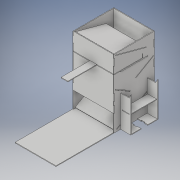
# Autodesk Inventor part: Full Tower
Saved by Autodesk Inventor 2017 (Build 210142000, 142)
## iProperties
Created: 2017-03-26
Part Number: Full Tower
Material: Generic
Document SubType Name: Modeling
Designer: Bearbiever
Density: 1 g/cm^3
Appearance: Default
Author: Bearbiever
Autodesk Inventor part; units mm, degrees
ref_plane "YZ Plane" through (0, 0, 0) normal (1, 0, 0) x (0, 1, 0)
ref_plane "XZ Plane" through (0, 0, 0) normal (0, 1, 0) x (-1, 0, 0)
ref_plane "XY Plane" through (0, 0, 0) normal (0, 0, 1) x (1, 0, 0)
sketch "Sketch15" plane through (0, 0, 0) normal (1, 0, 0) x (0, 1, 0)
  line L0 (254, 0) -> (254, 152.4)
  line L1 (190.4803, 152.4) -> (190.4803, 46.99)
  line L2 (195.0007, 142.6426) -> (201.7101, 142.6426) construction
  line L3 (201.7101, 142.6426) -> (201.7101, 48.7112) construction
  line L4 (201.7101, 48.7112) -> (195.0007, 48.7112) construction
  line L5 (195.0007, 48.7112) -> (195.0007, 142.6426) construction
  line L6 (190.4803, 152.4) -> (190.4803, 273.05)
  line L7 (6.35, 141.4015) -> (75.2882, 21.997)
  line L8 (136.614, 147.0706) -> (104.864, 92.078)
  line L9 (247.1811, 145.8462) -> (216.6784, 32.0086)
  line L10 (175.7069, 3.6254) -> (137.6069, 69.6166)
  line L11 (190.4803, 44.45) -> (203.1803, 44.45)
  line L12 (137.6069, 69.6166) -> (139.8066, 70.8866)
  line L13 (139.8066, 70.8866) -> (177.9066, 4.8954)
  line L14 (104.864, 92.078) -> (107.3637, 90.6348)
  line L15 (0, 152.4) -> (0.1917, 152.5107)
  line L16 (190.4803, 44.45) -> (187.9403, 44.45)
  line L17 (187.9403, 127) -> (187.9403, 273.05)
  line L18 (187.9403, 273.05) -> (190.4803, 273.05)
  line L19 (203.1803, 44.45) -> (203.1803, 46.99)
  line L20 (203.1803, 46.99) -> (190.4803, 46.99)
  line L21 (216.6784, 32.0086) -> (219.1318, 31.3512)
  line L22 (219.1318, 31.3512) -> (249.6345, 145.1888)
  line L23 (187.9403, 127) -> (185.4003, 127)
  line L24 (185.4003, 127) -> (185.4003, 25.4)
  line L25 (185.4003, 25.4) -> (187.9403, 25.4)
  line L26 (187.9403, 25.4) -> (187.9403, 44.45)
  line L27 (254, 0) -> (228.6, 0)
  line L28 (228.6, 0) -> (228.6, 2.54)
  line L29 (228.6, 2.54) -> (203.2, 2.54)
  line L30 (203.2, 2.54) -> (203.2, 0)
  line L31 (165.1, 0) -> (165.1, 2.54)
  line L32 (165.1, 2.54) -> (139.7, 2.54)
  line L33 (139.7, 2.54) -> (139.7, 0)
  line L34 (139.7, 0) -> (76.2, 0)
  line L35 (76.2, 0) -> (76.2, 2.54)
  line L36 (76.2, 2.54) -> (50.8, 2.54)
  line L37 (50.8, 2.54) -> (50.8, 0)
  line L38 (228.6, 0) -> (254, 0)
  line L39 (76.2, 0) -> (139.7, 0)
  line L40 (254, 152.4) -> (241.3, 152.4)
  line L41 (241.3, 152.4) -> (241.3, 149.86)
  line L42 (241.3, 149.86) -> (215.9, 149.86)
  line L43 (215.9, 149.86) -> (215.9, 152.4)
  line L44 (254, 152.4) -> (241.3, 152.4)
  line L45 (127, 152.4) -> (127, 149.86)
  line L46 (127, 149.86) -> (101.6, 149.86)
  line L47 (101.6, 149.86) -> (101.6, 152.4)
  line L48 (101.6, 152.4) -> (88.9, 152.4)
  line L49 (88.9, 152.4) -> (88.9, 149.86)
  line L50 (88.9, 149.86) -> (63.5, 149.86)
  line L51 (63.5, 149.86) -> (63.5, 152.4)
  line L52 (63.5, 152.4) -> (38.1, 152.4)
  line L53 (63.5, 152.4) -> (0, 152.4)
  line L54 (101.6, 152.4) -> (88.9, 152.4)
  line L55 (0, 152.4) -> (0, 127)
  line L56 (0, 127) -> (2.54, 127)
  line L57 (2.54, 127) -> (2.54, 88.9)
  line L58 (2.54, 88.9) -> (0, 88.9)
  line L59 (0, 88.9) -> (0, 63.5)
  line L60 (0, 63.5) -> (2.54, 63.5)
  line L61 (2.54, 63.5) -> (2.54, 25.4)
  line L62 (2.54, 25.4) -> (0, 25.4)
  line L63 (0, 152.4) -> (0, 127)
  line L64 (0, 88.9) -> (0, 63.5)
  line L65 (75.2882, 21.997) -> (77.4879, 23.267)
  line L66 (8.5497, 142.6715) -> (6.35, 141.4015)
  line L67 (8.5497, 142.6715) -> (77.4879, 23.267)
  line L68 (139.1137, 145.6275) -> (107.3637, 90.6348)
  line L69 (177.9066, 4.8954) -> (175.7069, 3.6254)
  line L70 (247.1811, 145.8462) -> (249.6345, 145.1888)
  line L71 (136.614, 147.0706) -> (139.1137, 145.6275)
  line L72 (127, 152.4) -> (187.9403, 152.4)
  line L73 (0, 25.4) -> (0, 0)
  line L74 (0, 0) -> (50.8, 0)
  line L75 (215.9, 152.4) -> (190.4803, 152.4)
  line L76 (203.2, 0) -> (165.1, 0)
  dimension "d39" = 254
  dimension "d40" = 152.4
  dimension "d42" = 120.65
  dimension "d49" = 12.7
  dimension "d53" = 2.54
  dimension "d56" = 2.54
  dimension "d57" = 2.54
  dimension "d58" = 2.54
  dimension "d59" = 2.54
  dimension "d60" = 101.6
  dimension "d62" = 25.4
  dimension "d65" = 2.54
  dimension "d66" = 25.4
  dimension "d67" = 38.1
  dimension "d68" = 2.54
  dimension "d69" = 25.4
  dimension "d70" = 63.5
  dimension "d71" = 2.54
  dimension "d72" = 25.4
  dimension "d73" = 12.7
  dimension "d74" = 2.54
  dimension "d75" = 25.4
  dimension "d80" = 2.54
  dimension "d81" = 25.4
  dimension "d82" = 12.7
  dimension "d83" = 2.54
  dimension "d84" = 25.4
  dimension "d85" = 25.4
  dimension "d86" = 25.4
  dimension "d87" = 2.54
  dimension "d88" = 38.1
  dimension "d89" = 25.4
  dimension "d90" = 2.54
  dimension "d91" = 38.1
  dimension "d94" = 6.35
  dimension "d95" = 30
  dimension "d96" = 76.2
  dimension "d98" = 63.5
  dimension "d99" = 25.4
  dimension "d100" = 50.8
  dimension "d101" = 2.54
  dimension "d102" = 2.54
  dimension "d103" = 2.54
  constraints: 154 end point, 47 perpendicular, 14 parallel, 9 horizontal, 7 point on line, 5 vertical
  measures "d39" distance of L15.start L0.end
  measures "d40" distance of L0.end L0.start
  measures "d42" distance of L1.start L6.end
  measures "d49" distance of L11.start L11.end
  measures "d53" distance of L10.end L12.end
  measures "d56" distance of L16.end L11.start
  measures "d57" distance of L11.end L19.end
  measures "d58" distance of L9.end L21.end
  measures "d59" distance of L25.end L24.end
  measures "d60" distance of L24.end L23.end
  measures "d62" distance of L0.start L27.end
  measures "d65" distance of L27.end L28.end
  measures "d66" distance of L28.end L29.end
  measures "d67" distance of L30.end L31.start
  measures "d68" distance of L31.start L31.end
  measures "d69" distance of L31.end L32.end
  measures "d70" distance of L33.end L34.end
  measures "d71" distance of L34.end L35.end
  measures "d72" distance of L35.end L36.end
  measures "d73" distance of L0.end L40.end
  measures "d74" distance of L40.end L41.end
  measures "d75" distance of L41.end L42.end
  measures "d80" distance of L45.start L45.end
  measures "d81" distance of L45.end L46.end
  measures "d82" distance of L47.end L48.end
  measures "d83" distance of L48.end L49.end
  measures "d84" distance of L49.end L50.end
  measures "d85" distance of L51.end L52.end
  measures "d86" distance of L15.start L55.end
  measures "d87" distance of L55.end L56.end
  measures "d88" distance of L56.end L57.end
  measures "d89" distance of L58.end L59.end
  measures "d90" distance of L59.end L60.end
  measures "d91" distance of L60.end L61.end
  measures "d94" distance from line of L55 L7.start
  measures "d95" angle of L55 L7
  measures "d96" distance between parallel lines of L69 L12
  measures "d98" distance between parallel lines of L14 L71
  measures "d99" distance of L73.end L62.end
  measures "d100" distance of L73.end L37.end
  measures "d101" distance of L61.end L62.end
  measures "d102" distance of L36.end L37.end
  measures "d103" distance of L32.end L33.end
extrude "Extrusion10" add sketch "Sketch15" along normal blind 2.54 contours L27 L28 L29 L30 L76 L31 L32 L33 L34 L35 L36 L37 L74 L73 L62 L61 L60 L59 L58 L57 L56 L55 L53 L52 L51 L50 L49 L48 L47 L46 L45 L72 L17 L23 L24 L25 L26 L16 L11 L19 L20 L1 L75 L43 L42 L41 L40 L0
sketch "Sketch16" plane through (0, 0, 0) normal (0, 0, -1) x (-1, 0, 0)
  line L0 (0, 0) -> (147.32, 0)
  line L1 (0, 0) -> (0, 50.8)
  line L2 (0, 50.8) -> (-2.54, 50.8)
  line L3 (-2.54, 50.8) -> (-2.54, 76.2)
  line L4 (-2.54, 76.2) -> (0, 76.2)
  line L5 (0, 139.7) -> (-2.54, 139.7) projected
  line L6 (0, 76.2) -> (0, 139.7)
  line L7 (0, 139.7) -> (-2.54, 139.7)
  line L8 (0, 165.1) -> (-2.54, 165.1) projected
  line L9 (-2.54, 139.7) -> (-2.54, 165.1)
  line L10 (-2.54, 165.1) -> (0, 165.1)
  line L11 (0, 165.1) -> (0, 203.2) projected
  line L12 (0, 165.1) -> (0, 203.2)
  line L13 (0, 203.2) -> (-2.54, 203.2)
  line L14 (-2.54, 203.2) -> (-2.54, 228.6) projected
  line L15 (-2.54, 203.2) -> (-2.54, 228.6)
  line L16 (-2.54, 228.6) -> (0, 228.6)
  line L17 (0, 254) -> (-2.54, 254) projected
  line L18 (0, 228.6) -> (0, 254)
  line L19 (0, 254) -> (147.32, 254)
  line L20 (147.32, 0) -> (147.32, 50.8)
  line L21 (147.32, 50.8) -> (149.86, 50.8)
  line L22 (149.86, 50.8) -> (149.86, 76.2)
  line L23 (149.86, 76.2) -> (147.32, 76.2)
  line L24 (147.32, 76.2) -> (147.32, 139.7)
  line L25 (147.32, 139.7) -> (149.86, 139.7)
  line L26 (149.86, 139.7) -> (149.86, 165.1)
  line L27 (149.86, 165.1) -> (147.32, 165.1)
  line L28 (147.32, 165.1) -> (147.32, 203.2)
  line L29 (147.32, 203.2) -> (149.86, 203.2)
  line L30 (149.86, 203.2) -> (149.86, 228.6)
  line L31 (149.86, 228.6) -> (147.32, 228.6)
  line L32 (147.32, 228.6) -> (147.32, 254)
  dimension "d106" = 147.32
  dimension "d107" = 147.32
  dimension "d108" = 50.8
  dimension "d109" = 2.54
  dimension "d110" = 25.4
  dimension "d111" = 2.54
  constraints: 56 end point, 18 perpendicular, 12 point on line, 2 vertical, 1 horizontal
  measures "d106" distance of L0.start L0.end
  measures "d107" distance of L17.start L19.end
  measures "d108" distance of L0.end L20.end
  measures "d109" distance of L20.end L21.end
  measures "d110" distance of L21.end L22.end
  measures "d111" distance of L24.end L25.end
extrude "Extrusion11" add sketch "Sketch16" against normal blind 2.54 separate body
sketch "Sketch19" plane through (-149.86, 203.2, 0) normal (-1, 0, 0) x (0, 0, 1)
  line L0 (0, 50.8) -> (152.4, 50.8) projected
  line L1 (152.4, 50.8) -> (0, 50.8)
  line L2 (0, 0) -> (0, 25.4) projected
  line L3 (0, 50.8) -> (0, 25.4)
  line L4 (2.54, 50.8) -> (2.54, 25.4) projected
  line L5 (0, 25.4) -> (2.54, 25.4)
  line L6 (2.54, 25.4) -> (2.54, 0)
  line L7 (2.54, 0) -> (0, 0)
  line L8 (0, -38.1) -> (0, -63.5) projected
  line L9 (0, 0) -> (0, -38.1)
  line L10 (0, -38.1) -> (2.54, -38.1)
  line L11 (2.54, -127) -> (2.54, -63.5) projected
  line L12 (2.54, -38.1) -> (2.54, -63.5)
  line L13 (2.54, -63.5) -> (0, -63.5)
  line L14 (0, -127) -> (0, -152.4) projected
  line L15 (0, -63.5) -> (0, -127)
  line L16 (2.54, -152.4) -> (2.54, -127) projected
  line L17 (2.54, -127) -> (2.54, -152.4)
  line L18 (2.54, -152.4) -> (0, -152.4)
  line L19 (0, -203.2) -> (25.4, -203.2)
  line L20 (63.5, -200.66) -> (25.4, -200.66) projected
  line L21 (25.4, -203.2) -> (25.4, -200.66)
  line L22 (25.4, -200.66) -> (63.5, -200.66)
  line L23 (63.5, -200.66) -> (63.5, -203.2)
  line L24 (63.5, -203.2) -> (88.9, -203.2)
  line L25 (88.9, -203.2) -> (88.9, -200.66)
  line L26 (127, -203.2) -> (127, -200.66) projected
  line L27 (88.9, -200.66) -> (127, -200.66)
  line L28 (127, -200.66) -> (127, -203.2)
  line L29 (127, -203.2) -> (152.4, -203.2)
  line L30 (152.4, -203.2) -> (152.4, -139.7)
  line L31 (149.86, -139.7) -> (152.4, -139.7) projected
  line L32 (152.4, -139.7) -> (149.86, -139.7)
  line L33 (149.86, -139.7) -> (149.86, -114.3)
  line L34 (152.4, -101.6) -> (152.4, -114.3) projected
  line L35 (149.86, -114.3) -> (152.4, -114.3)
  line L36 (152.4, -114.3) -> (152.4, -101.6)
  line L37 (152.4, -101.6) -> (149.86, -101.6)
  line L38 (152.4, -76.2) -> (149.86, -76.2) projected
  line L39 (149.86, -101.6) -> (149.86, -76.2)
  line L40 (149.86, -76.2) -> (152.4, -76.2)
  line L41 (127, -15.2597) -> (152.4, -15.2597) projected
  line L42 (152.4, -76.2) -> (152.4, -15.2597)
  line L43 (152.4, -15.2597) -> (127, -15.2597)
  line L44 (25.4, -17.7997) -> (127, -17.7997) projected
  line L45 (127, -15.2597) -> (127, -17.7997)
  line L46 (127, -17.7997) -> (25.4, -17.7997)
  line L47 (25.4, -17.7997) -> (25.4, -15.2597)
  line L48 (25.4, -15.2597) -> (44.45, -15.2597)
  line L49 (44.45, -0.0197) -> (44.45, -15.2597) projected
  line L50 (44.45, -15.2597) -> (44.45, -0.0197)
  line L51 (44.45, -0.0197) -> (46.99, -0.0197)
  line L52 (46.99, -12.7197) -> (46.99, -0.0197) projected
  line L53 (46.99, -0.0197) -> (46.99, -12.7197)
  line L54 (152.4, 12.7) -> (152.4, -12.7197) projected
  line L55 (46.99, -12.7197) -> (152.4, -12.7197)
  line L56 (152.4, -12.7197) -> (152.4, 12.7)
  line L57 (149.86, 12.7) -> (152.4, 12.7) projected
  line L58 (152.4, 12.7) -> (149.86, 12.7)
  line L59 (149.86, 12.7) -> (149.86, 38.1)
  line L60 (149.86, 38.1) -> (152.4, 38.1)
  line L61 (152.4, 38.1) -> (152.4, 50.8)
  line L62 (31.3512, 15.9318) -> (145.1888, 46.4345)
  line L63 (145.1888, 46.4345) -> (145.8462, 43.9811)
  line L64 (31.3512, 15.9318) -> (32.0086, 13.4784) projected
  line L65 (145.8462, 43.9811) -> (32.0086, 13.4784)
  line L66 (32.0086, 13.4784) -> (31.3512, 15.9318)
  line L67 (4.8954, -25.2934) -> (70.8866, -63.3934) projected
  line L68 (4.8954, -25.2934) -> (70.8866, -63.3934)
  line L69 (70.8866, -63.3934) -> (69.6166, -65.5931) projected
  line L70 (70.8866, -63.3934) -> (69.6166, -65.5931)
  line L71 (69.6166, -65.5931) -> (3.6254, -27.4931) projected
  line L72 (69.6166, -65.5931) -> (3.6254, -27.4931)
  line L73 (3.6254, -27.4931) -> (4.8954, -25.2934) projected
  line L74 (3.6254, -27.4931) -> (4.8954, -25.2934)
  line L75 (147.0706, -66.586) -> (145.6275, -64.0863) projected
  line L76 (145.6275, -64.0863) -> (147.0706, -66.586)
  line L77 (147.0706, -66.586) -> (92.078, -98.336)
  line L78 (92.078, -98.336) -> (90.6348, -95.8363)
  line L79 (90.6348, -95.8363) -> (145.6275, -64.0863)
  line L80 (23.267, -125.7121) -> (142.6715, -194.6503) projected
  line L81 (23.267, -125.7121) -> (21.997, -127.9118)
  line L82 (141.4015, -196.85) -> (21.997, -127.9118) projected
  line L83 (21.997, -127.9118) -> (141.4015, -196.85)
  line L84 (141.4015, -196.85) -> (142.6715, -194.6503)
  line L85 (142.6715, -194.6503) -> (23.267, -125.7121)
  line L86 (0, -152.4) -> (0, -203.2)
  dimension "d157" = 25.4
  dimension "d158" = 2.54
  dimension "d159" = 2.54
  constraints: 122 end point, 41 perpendicular, 12 collinear, 11 point on line, 2 horizontal, 2 vertical
  measures "d157" distance of L31.start L33.end
  measures "d158" distance of L62.end L63.end
  measures "d159" distance of L67.end L69.end
extrude "Extrusion12" add sketch "Sketch19" against normal blind 2.54 separate body contours L0 L4 L5 L3 | L0 L61 L60 L59 L57 L54 L55 L52 L51 L49 L48 L47 L44 L45 L41 L42 L38 L39 L37 L34 L35 L33 L31 L30 L29 L26 L27 L25 L24 L23 L20 L21 L19 L86 L18 L16 L11 L12 L10 L9 L7 L6 L4
sketch "Sketch20" plane through (-149.86, 187.9403, 152.4) normal (0, 1, 0) x (1, 0, 0)
  line L0 (152.4, 127) -> (152.4, 25.4) projected
  line L1 (0, 0) -> (0, 107.95)
  line L2 (0, 107.95) -> (152.4, 107.95)
  line L3 (152.4, 107.95) -> (152.4, 0)
  line L4 (88.9, 0) -> (88.9, -107.95)
  line L5 (88.9, -107.95) -> (63.5, -107.95)
  line L6 (63.5, -107.95) -> (63.5, 0)
  line L7 (152.4, 0) -> (88.9, 0)
  line L8 (63.5, 0) -> (0, 0)
  point P0 (149.86, 152.4)
  dimension "d163" = 107.95
  dimension "d164" = 152.4
  dimension "d165" = 107.95
  dimension "d166" = 25.4
  dimension "d167" = 63.5
  constraints: 16 end point, 8 perpendicular, 1 point on line, 1 vertical
  measures "d163" distance of L1.start L1.end
  measures "d164" distance of L1.end L2.end
  measures "d165" distance of L4.start L4.end
  measures "d166" distance of L4.end L5.end
  measures "d167" distance of L1.start L6.end
extrude "Extrusion13" add sketch "Sketch20" along normal blind 2.54 separate body
sketch "Sketch21" plane through (0, 187.9403, 44.45) normal (0, 0, 1) x (1, 0, 0)
  line L0 (2.54, 15.24) -> (2.54, 0) projected
  line L1 (2.54, 2.5499) -> (-149.86, 2.5499)
  line L2 (-149.86, 2.5499) -> (-149.86, 15.2499)
  line L3 (-149.86, 15.2499) -> (2.54, 15.2499)
  line L4 (2.54, 15.2499) -> (2.54, 2.5499)
  point P0 (0, -187.9403)
  dimension "d170" = 152.4
  dimension "d171" = 12.7
  constraints: 8 end point, 2 parallel, 1 horizontal, 1 perpendicular, 1 point on line
  measures "d170" distance of L2.end L3.end
  measures "d171" distance of L1.end L2.end
extrude "Extrusion14" add sketch "Sketch21" along normal blind 2.54 separate body
sketch "Sketch23" plane through (-149.86, 241.3, 152.4) normal (0, 0, 1) x (1, 0, 0)
  line L0 (149.86, 12.7) -> (149.86, 0) projected
  line L1 (2.54, 12.7) -> (149.86, 12.7)
  line L2 (149.86, 12.7) -> (149.86, 0)
  line L3 (149.86, 0) -> (152.4, 0)
  line L4 (152.4, 0) -> (152.4, -25.4)
  line L5 (152.4, -25.4) -> (149.86, -25.4)
  line L6 (149.86, -114.3) -> (152.4, -114.3) projected
  line L7 (149.86, -25.4) -> (149.86, -114.3)
  line L8 (149.86, -114.3) -> (152.4, -114.3)
  line L9 (152.4, -114.3) -> (152.4, -139.7)
  line L10 (149.86, -139.7) -> (149.86, -152.4) projected
  line L11 (152.4, -139.7) -> (149.86, -139.7)
  line L12 (149.86, -139.7) -> (149.86, -152.4)
  line L13 (149.86, -152.4) -> (152.4, -152.4) projected
  line L14 (149.86, -152.4) -> (152.4, -152.4)
  line L15 (152.4, -177.8) -> (152.4, -241.3) projected
  line L16 (152.4, -152.4) -> (152.4, -177.8)
  line L17 (149.86, -177.8) -> (149.86, -241.3) projected
  line L18 (152.4, -177.8) -> (149.86, -177.8)
  line L19 (2.54, -177.8) -> (0, -177.8)
  line L20 (0, -177.8) -> (0, -152.4)
  line L21 (0, -152.4) -> (2.54, -152.4)
  line L22 (2.54, -152.4) -> (2.54, -139.7)
  line L23 (2.54, -139.7) -> (0, -139.7)
  line L24 (0, -114.3) -> (0, -53.3597) projected
  line L25 (0, -139.7) -> (0, -114.3)
  line L26 (0, -114.3) -> (2.54, -114.3)
  line L27 (2.54, -25.4) -> (2.54, -50.8197) projected
  line L28 (2.54, -114.3) -> (2.54, -25.4)
  line L29 (2.54, -25.4) -> (0, -25.4)
  line L30 (0, 0) -> (0, 12.7) projected
  line L31 (0, -25.4) -> (0, 0)
  line L32 (0, 0) -> (2.54, 0)
  line L33 (2.54, 0) -> (2.54, 12.7)
  line L34 (63.5, -53.3597) -> (63.5, -50.8197) projected
  line L35 (88.9, -50.8197) -> (152.4, -50.8197) projected
  line L36 (63.5, -53.3597) -> (88.9, -53.3597)
  line L37 (88.9, -53.3597) -> (88.9, -50.8197)
  line L38 (88.9, -50.8197) -> (63.5, -50.8197)
  line L39 (63.5, -50.8197) -> (63.5, -53.3597)
  line L40 (2.54, -177.8) -> (149.86, -177.8)
  point P0 (149.86, -196.85)
  dimension "d175" = 2.54
  dimension "d176" = 19.05
  constraints: 60 end point, 18 perpendicular, 4 point on line, 2 collinear, 2 horizontal, 2 parallel
  measures "d175" distance of L0.end L3.end
  measures "d176" distance of L17.start point (149.86, -196.85)
sketch "Sketch22" plane through (0, 247.1811, 145.8462) normal (0, 0.9659258, -0.258819) x (1, 0, 0)
  line L0 (0, 117.8533) -> (2.54, 117.8533) projected
  line L1 (0, 0) -> (2.54, 0) projected
  line L2 (2.54, 0) -> (-149.86, 0)
  line L3 (-149.86, 0) -> (-149.86, 117.8533)
  line L4 (-149.86, 117.8533) -> (2.54, 117.8533)
  line L5 (2.54, 117.8533) -> (2.54, 0)
  point P0 (0, 204.8517)
  dimension "d174" = 152.4
  constraints: 8 end point, 2 parallel, 1 horizontal, 1 perpendicular
  measures "d174" distance of L3.end L4.end
extrude "Extrusion15" add sketch "Sketch22" along normal blind 2.54 separate body
extrude "Extrusion16" add sketch "Sketch23" against normal blind 2.54 separate body
sketch "Sketch24" plane through (-149.86, 177.9066, 4.8954) normal (0, -0.8660254, -0.5) x (1, 0, 0)
  line L0 (0, 0) -> (2.54, 0) projected
  line L1 (0, 76.2) -> (2.54, 76.2) projected
  line L2 (0, 0) -> (0, 76.2)
  line L3 (152.4, 76.2) -> (152.4, 0) projected
  line L4 (0, 76.2) -> (152.4, 76.2)
  line L5 (0, 30.1632) -> (152.4, 30.1632) projected
  line L6 (152.4, 76.2) -> (152.4, 0)
  line L7 (2.54, 0) -> (2.54, -2.1623)
  line L8 (2.54, -2.1623) -> (149.86, -2.1623)
  line L9 (149.86, -2.1623) -> (149.86, 0)
  line L10 (0, 0) -> (2.54, 0)
  line L11 (149.86, 0) -> (152.4, 0)
  point P0 (149.86, 84.7137)
  dimension "d182" = 152.4
  dimension "d183" = 152.4
  dimension "d184" = 147.32
  constraints: 16 end point, 5 perpendicular, 3 vertical, 1 parallel
  measures "d182" distance of L0.start L3.end
  measures "d183" distance of L1.start L3.start
  measures "d184" distance of L7.end L8.end
extrude "Extrusion17" add sketch "Sketch24" along normal blind 2.54 separate body
sketch "Sketch25" plane through (-149.86, 107.3637, 90.6348) normal (0, -0.8660254, 0.5) x (1, 0, 0)
  line L0 (152.4, 63.5) -> (152.4, 0) projected
  line L1 (152.4, 0) -> (152.4, 63.5)
  line L2 (152.4, 0) -> (0, 0)
  line L3 (0, 63.5) -> (2.54, 63.5) projected
  line L4 (0, 0) -> (0, 63.5)
  line L5 (149.86, 63.5) -> (149.86, 66.04)
  line L6 (149.86, 66.04) -> (2.54, 66.04)
  line L7 (2.54, 66.04) -> (2.54, 63.5)
  line L8 (0, 63.5) -> (2.54, 63.5)
  line L9 (149.86, 63.5) -> (152.4, 63.5)
  point P0 (149.86, -132.1739)
  dimension "d187" = 152.4
  dimension "d188" = 152.4
  dimension "d189" = 2.54
  dimension "d190" = 147.32
  constraints: 16 end point, 2 perpendicular, 1 collinear, 1 horizontal, 1 vertical
  measures "d187" distance of L0.end L2.end
  measures "d188" distance of L3.start L0.start
  measures "d189" distance of L5.start L5.end
  measures "d190" distance of L5.end L6.end
extrude "Extrusion18" add sketch "Sketch25" along normal blind 2.54 separate body
sketch "Sketch26" plane through (0, 6.35, 141.4015) normal (0, 0.8660254, 0.5) x (1, 0, 0)
  line L0 (2.54, 137.8764) -> (2.54, 0) projected
  line L1 (2.54, 0) -> (2.54, 137.8764)
  line L2 (-149.86, 0) -> (-149.86, 137.8764) projected
  line L3 (-149.86, 0) -> (-149.86, 137.8764)
  line L4 (-149.86, 137.8764) -> (-147.32, 137.8764) projected
  line L5 (-149.86, 137.8764) -> (-147.32, 137.8764)
  line L6 (2.54, 137.8764) -> (0, 137.8764)
  line L7 (0, 137.8764) -> (0, 158.1964)
  line L8 (0, 158.1964) -> (-147.32, 158.1964)
  line L9 (-147.32, 158.1964) -> (-147.32, 137.8764)
  line L10 (-149.86, 0) -> (-147.32, 0) projected
  line L11 (-149.86, 0) -> (-147.32, 0)
  line L12 (-147.32, 0) -> (-147.32, -5.08)
  line L13 (-147.32, -5.08) -> (0, -5.08)
  line L14 (0, -5.08) -> (0, 0)
  line L15 (2.54, 0) -> (0, 0)
  line L16 (-147.32, 0) -> (-149.86, 0)
  dimension "d195" = 20.32
  dimension "d196" = 147.32
  dimension "d197" = 5.08
  dimension "d198" = 147.32
  constraints: 26 end point, 3 collinear, 3 horizontal, 3 perpendicular, 2 parallel, 2 vertical
  measures "d195" distance of L6.end L7.end
  measures "d196" distance of L7.end L8.end
  measures "d197" distance of L10.end L12.end
  measures "d198" distance of L12.end L13.end
extrude "Extrusion19" add sketch "Sketch26" along normal blind 2.54 separate body
sketch "Sketch29" plane through (-149.86, 0, 0) normal (0, -1, 0) x (1, 0, 0)
  line L0 (2.54, 2.54) -> (149.86, 2.54) projected
  line L1 (2.54, 2.54) -> (149.86, 2.54)
  line L2 (149.86, 25.4) -> (149.86, 0) projected
  line L3 (149.86, 2.54) -> (149.86, 25.4)
  line L4 (149.86, 88.9) -> (149.86, 63.5) projected
  line L5 (149.86, 63.5) -> (149.86, 88.9)
  line L6 (149.86, 152.4) -> (149.86, 127) projected
  line L7 (149.86, 127) -> (149.86, 152.4)
  line L8 (149.86, 152.4) -> (152.4, 152.4)
  line L9 (152.4, 152.4) -> (152.4, 368.3)
  line L10 (152.4, 368.3) -> (0, 368.3)
  line L11 (0, 368.3) -> (0, 152.4)
  line L12 (0, 63.5) -> (2.54, 63.5) projected
  line L13 (2.54, 88.9) -> (2.54, 63.5) projected
  line L14 (2.54, 63.5) -> (2.54, 88.9)
  line L15 (2.54, 63.5) -> (0, 63.5)
  line L16 (0, 25.4) -> (2.54, 25.4)
  line L17 (2.54, 25.4) -> (0, 25.4)
  line L18 (0, 152.4) -> (2.54, 152.4)
  line L19 (2.54, 152.4) -> (2.54, 127)
  line L20 (0, 88.9) -> (2.54, 88.9) projected
  line L21 (0, 88.9) -> (2.54, 88.9)
  line L22 (0, 63.5) -> (0, 25.4)
  line L23 (2.54, 25.4) -> (2.54, 2.54)
  line L24 (0, 88.9) -> (0, 127)
  line L25 (0, 127) -> (2.54, 127) projected
  line L26 (0, 127) -> (2.54, 127)
  line L27 (0, 127) -> (2.54, 127) projected
  line L28 (149.86, 127) -> (152.4, 127) projected
  line L29 (149.86, 127) -> (190.5, 127)
  line L30 (190.5, 127) -> (190.5, 88.9)
  line L31 (190.5, 88.9) -> (149.86, 88.9)
  line L32 (149.86, 63.5) -> (190.5, 63.5)
  line L33 (190.5, 63.5) -> (190.5, 25.4)
  line L34 (190.5, 25.4) -> (149.86, 25.4)
  dimension "d221" = 40.64
  dimension "d222" = 38.1
  constraints: 50 end point, 7 collinear, 6 perpendicular, 3 horizontal, 3 point on line, 3 vertical, 1 parallel
  measures "d221" distance of L6.end L29.end
  measures "d222" distance of L29.end L30.end
extrude "Extrusion20" add sketch "Sketch29" against normal blind 2.54 separate body
sketch "Sketch31" plane through (-149.86, 2.54, 0) normal (0, 1, 0) x (1, 0, 0)
  line L0 (177.8, -127) -> (177.8, -124.46)
  line L1 (177.8, -124.46) -> (165.1, -124.46)
  line L2 (165.1, -124.46) -> (165.1, -127)
  line L3 (177.8, -127) -> (165.1, -127)
  line L4 (177.8, -88.9) -> (177.8, -91.44)
  line L5 (177.8, -91.44) -> (165.1, -91.44)
  line L6 (165.1, -91.44) -> (165.1, -88.9)
  point P0 (149.86, 0)
  dimension "d224" = 2.54
  dimension "d225" = 12.7
  dimension "d226" = 2.54
  dimension "d228" = 2.54
  dimension "d229" = 12.7
  constraints: 14 end point, 2 perpendicular, 1 horizontal, 1 vertical
  measures "d224" distance of L0.start L0.end
  measures "d225" distance of L0.end L1.end
  measures "d226" distance of L1.end L2.end
  measures "d228" distance of L4.start L4.end
  measures "d229" distance of L4.end L5.end
extrude "Extrusion21" cut sketch "Sketch31" against normal blind 2.54 bodies 11
sketch "Sketch32" plane through (-149.86, 2.54, 0) normal (0, 1, 0) x (1, 0, 0)
  line L0 (177.8, -88.9) -> (177.8, -91.44)
  line L1 (177.8, -91.44) -> (165.1, -91.44)
  line L2 (165.1, -91.44) -> (165.1, -88.9)
  line L3 (177.8, -88.9) -> (165.1, -88.9)
  point P0 (149.86, 0)
  dimension "d233" = 2.54
  dimension "d234" = 12.7
  constraints: 8 end point, 2 perpendicular, 1 horizontal
  measures "d233" distance of L0.start L0.end
  measures "d234" distance of L0.end L1.end
extrude "Extrusion22" cut sketch "Sketch32" against normal blind 2.54 bodies 11
sketch "Sketch33" plane through (-149.86, 2.54, 0) normal (0, 1, 0) x (1, 0, 0)
  line L0 (177.8, -63.5) -> (177.8, -60.96)
  line L1 (177.8, -60.96) -> (165.1, -60.96)
  line L2 (165.1, -60.96) -> (165.1, -63.5)
  line L3 (165.1, -63.5) -> (177.8, -63.5)
  point P0 (149.86, 0)
  dimension "d238" = 2.54
  dimension "d239" = 12.7
  dimension "d240" = 2.54
  constraints: 8 end point, 1 horizontal, 1 perpendicular
  measures "d238" distance of L0.start L0.end
  measures "d239" distance of L0.end L1.end
  measures "d240" distance of L1.end L2.end
extrude "Extrusion23" cut sketch "Sketch33" against normal blind 2.54 bodies 11
sketch "Sketch34" plane through (-149.86, 2.54, 0) normal (0, 1, 0) x (1, 0, 0)
  line L0 (190.5, -25.4) -> (190.5, -63.5) projected
  line L1 (177.8, -25.4) -> (177.8, -27.94)
  line L2 (177.8, -27.94) -> (165.1, -27.94)
  line L3 (165.1, -27.94) -> (165.1, -25.4)
  line L4 (165.1, -25.4) -> (177.8, -25.4)
  line L5 (149.86, -25.4) -> (190.5, -25.4) projected
  point P0 (149.86, 0)
  dimension "d244" = 2.54
  dimension "d245" = 12.7
  constraints: 8 end point, 2 perpendicular, 1 collinear, 1 vertical
  measures "d244" distance of L1.start L1.end
  measures "d245" distance of L1.end L2.end
extrude "Extrusion24" cut sketch "Sketch34" against normal blind 2.54 bodies 11
sketch "Sketch35" plane through (0, 0, 127) normal (0, 0, 1) x (1, 0, 0)
  line L0 (27.94, 2.54) -> (40.64, 2.54) projected
  line L1 (40.64, 2.54) -> (27.94, 2.54)
  line L2 (27.94, 2.54) -> (27.94, 0)
  line L3 (27.94, 0) -> (15.24, 0) projected
  line L4 (27.94, 0) -> (15.24, 0)
  line L5 (15.24, 2.54) -> (15.24, 0) projected
  line L6 (15.24, 0) -> (15.24, 2.54)
  line L7 (15.24, 2.54) -> (2.5375, 2.54)
  line L8 (0, 2.54) -> (15.24, 2.54) projected
  line L9 (40.64, 2.54) -> (40.64, 129.54)
  line L10 (2.5375, 2.54) -> (2.54, 116.84)
  line L11 (2.54, 116.84) -> (34.29, 116.8393)
  line L12 (34.29, 116.8393) -> (40.64, 129.54)
  line L13 (8.89, 66.04) -> (34.29, 66.04)
  line L14 (34.29, 66.04) -> (34.29, 63.5)
  line L15 (34.29, 63.5) -> (8.89, 63.5)
  line L16 (8.89, 63.5) -> (8.89, 66.04)
  point P0 (0, 0)
  dimension "d248" = 12.7
  dimension "d249" = 127
  dimension "d250" = 114.3
  dimension "d251" = 31.75
  dimension "d254" = 25.4
  dimension "d255" = 2.54
  dimension "d256" = 63.5
  dimension "d257" = 6.35
  constraints: 26 end point, 5 equal length, 3 perpendicular, 1 horizontal, 1 point on line, 1 vertical
  measures "d248" distance of L0.end L0.start
  measures "d249" distance of L0.end L9.end
  measures "d250" distance of L7.end L10.end
  measures "d251" distance of L10.end L11.end
  measures "d254" distance of L14.end L15.end
  measures "d255" distance of L13.end L14.end
  measures "d256" distance between parallel lines of L3 L15
  measures "d257" distance between parallel lines of L9 L14
extrude "Extrusion26" add sketch "Sketch35" against normal blind 2.54 bodies 11
sketch "Sketch37" plane through (40.64, 0, 25.4) normal (0, 0, -1) x (-1, 0, 0)
  line L0 (0, 0) -> (0, 2.54) projected
  line L1 (12.7, 2.54) -> (0, 2.54) projected
  line L2 (0, 2.54) -> (12.7, 2.54)
  line L3 (12.7, 2.54) -> (12.7, 0)
  line L4 (40.64, 0) -> (25.4, 0) projected
  line L5 (12.7, 0) -> (25.4, 0)
  line L6 (25.4, 2.54) -> (40.64, 2.54) projected
  line L7 (25.4, 0) -> (25.4, 2.54)
  line L8 (25.4, 2.54) -> (38.1, 2.54)
  line L9 (38.1, 116.8382) -> (38.1, 2.54)
  line L10 (38.1, 0) -> (38.1, 50.8) projected
  line L11 (0, 2.54) -> (0, 129.54)
  line L12 (38.1, 116.84) -> (6.35, 116.8393) projected
  line L13 (0, 129.54) -> (6.35, 116.8393)
  line L14 (6.35, 116.8393) -> (38.1, 116.84)
  line L15 (38.1, 116.84) -> (38.1, 2.54)
  line L16 (31.75, 66.04) -> (6.35, 66.04) projected
  line L17 (31.7483, 66.04) -> (6.35, 66.04)
  line L18 (6.35, 66.04) -> (6.35, 63.5) projected
  line L19 (6.35, 66.04) -> (6.35, 63.5)
  line L20 (31.75, 63.5) -> (31.75, 66.04) projected
  line L21 (6.35, 63.5) -> (31.75, 63.5)
  line L22 (31.75, 63.5) -> (31.75, 66.04)
  dimension "d260" = 127
  constraints: 28 end point, 5 perpendicular, 4 collinear, 2 horizontal, 2 point on line, 1 parallel
  measures "d260" distance of L0.end L11.end
extrude "Extrusion27" add sketch "Sketch37" against normal blind 2.54 contours L1 L11 L13 L12 L9 L6 L7 L5 L3 bodies 11
sketch "Sketch38" plane through (8.89, 63.5, 25.4) normal (0, 1, 0) x (1, 0, 0)
  line L0 (0, 0) -> (25.4, 0) projected
  line L1 (25.4, 0) -> (0, 0)
  line L2 (0, -101.6) -> (25.4, -101.6)
  line L3 (25.4, -2.54) -> (0, -2.54) projected
  line L4 (25.4, 0) -> (25.4, -2.54)
  line L5 (25.4, -2.54) -> (29.21, -2.54)
  line L6 (29.21, -2.54) -> (29.21, -99.06)
  line L7 (29.21, -99.06) -> (25.4, -99.06)
  line L8 (25.4, -101.6) -> (25.4, -99.06)
  line L9 (25.4, -2.54) -> (25.4, 0)
  line L10 (0, -99.06) -> (-3.81, -99.06)
  line L11 (-3.81, -99.06) -> (-3.81, -2.54)
  line L12 (-3.81, -2.54) -> (0, -2.54)
  line L13 (0, 0) -> (0, -2.54)
  line L14 (0, -99.06) -> (0, -101.6)
  point P0 (-8.89, 25.4)
  dimension "d263" = 2.54
  dimension "d264" = 3.81
  dimension "d265" = 96.52
  dimension "d266" = 3.81
  dimension "d267" = 96.52
  constraints: 26 end point, 11 perpendicular, 1 collinear, 1 horizontal, 1 vertical
  measures "d263" distance of L0.end L3.start
  measures "d264" distance of L3.start L5.end
  measures "d265" distance of L5.end L6.end
  measures "d266" distance of L10.start L10.end
  measures "d267" distance of L10.end L11.end
extrude "Extrusion28" add sketch "Sketch38" along normal blind 2.54 separate body contours L3 L5 L6 L7 L8 L2 L14 L10 L11 L12
body "Solid2"
body "Solid3"
body "Solid4"
body "Solid5"
body "Solid6"
body "Solid7"
body "Solid8"
body "Solid9"
body "Solid10"
body "Solid11"
body "Solid12"
body "Solid14"
